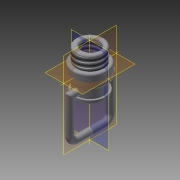
# Autodesk Inventor part: SchleppstangeBefestigungOben
Saved by Autodesk Inventor 2015 (Build 190159000, 159)
## iProperties
Created: 2018-11-19
Part Number: SchleppstangeBefestigungOben
Material: Generisch
Document SubType Name: Modeling
Designer: Boris
Density: 1 g/cm^3
Appearance: Vorgabe
Author: Boris
Autodesk Inventor part; units mm, degrees
sketch "Skizze1" plane through (0, 0, 0) normal (0, 0, 1) x (1, 0, 0)
  circle A0 centre (0, 0) radius 2.5
  dimension "d0" = 5
  constraints: 1 centre point, 1 coincident
  measures "d0" diameter of A0
extrude "Extrusion1" add sketch "Skizze1" along normal mid plane 2
sketch "Skizze2" plane through (0, 0, 0) normal (0, 0, 1) x (1, 0, 0)
  circle A0 centre (0, 0) radius 2
  dimension "d3" = 4
  constraints: 1 centre point, 1 coincident
  measures "d3" diameter of A0
extrude "Extrusion2" add sketch "Skizze2" along normal mid plane 6
hole "Bohrung1" at (0.0604, 0.0473, 3) direction (0, 0, -1) diameter 2.487 depth 3
fillet "Rundung1" radius 0.25 2 edges at (-2, 0, 3) (0.0604, 1.2908, 3)
thread "Gewinde1"
fillet "Rundung2" radius 0.25 2 edges at (-2.5, 0, 1) (-2.5, 0, -1)
sketch "Skizze3" plane through (0, 0, 0) normal (0, 1, 0) x (-1, 0, 0)
  circle A0 centre (0, -2) radius 0.5
  line L0 (2.25, -1) -> (-2.25, -1) projected
  point P0 (0, 0)
  dimension "d19" = 1
  dimension "d23" = 1
  constraints: 1 centre point
  measures "d19" diameter of A0
  measures "d23" distance from line of L0 A0.centre
sketch "Skizze4" plane through (0, 0, 0) normal (1, 0, 0) x (0, 1, 0)
  line L0 (2.25, -1) -> (-2.25, -1) projected
  line L1 (-3, -2) -> (3, -2)
  line L2 (3, -2) -> (3, -7)
  line L3 (2, -8) -> (-2, -8)
  line L4 (-3, -7) -> (-3, -2)
  line L5 (0, -10.2) -> (0, 5.2) projected
  arc A0 (-3, -7) -> (-2, -8) centre (-2, -7) ccw
  arc A1 (2, -8) -> (3, -7) centre (2, -7) ccw
  point P0 (0, 0)
  point P1 (3, -8)
  point P2 (-3, -8)
  dimension "d20" = 6
  dimension "d21" = 6
  dimension "d22" = 1
  dimension "d24" = 1
  constraints: 8 end point, 4 point on circle, 4 point on line, 4 tangent, 2 centre point, 2 parallel, 1 equal radius, 1 horizontal, 1 perpendicular, 1 other
  measures "d20" distance of point (3, -8) point (-3, -8)
  measures "d21" distance of L1.end point (3, -8)
  measures "d22" distance between parallel lines of L1 L0
  measures "d24" radius of A0
sweep "Sweeping1" add profiles "Skizze3" path "Skizze4" path curves L3 A0 L4 L1 L2 A1
sketch "Skizze5" plane through (0, 0, -3) normal (0, 0, -1) x (-1, 0, 0)
  circle A0 centre (0, 0) radius 2 projected
  circle A1 centre (0, 0) radius 2.25
  dimension "d27" = 4.5
  constraints: 1 centre point, 1 coincident
  measures "d27" diameter of A1
extrude "Extrusion3" add sketch "Skizze5" against normal blind 0.5
fillet "Rundung3" radius 0.125 1 edges at (2.25, 0, -3)
fillet "Rundung4" radius 0.125 1 edges at (-2, 0, -1)
